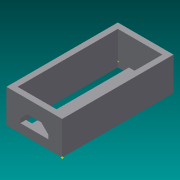
# Autodesk Inventor part: nano_enclosure
Saved by Autodesk Inventor 2015 (Build 190159000, 159)
## iProperties
Created: 2015-02-05
Part Number: nano_enclosure
Material: Generic
Document SubType Name: Modeling
Designer: Jeff
Density: 1 g/cm^3
Appearance: Default
Author: Jeff
Autodesk Inventor part; units mm, degrees
ref_plane "YZ Plane" through (0, 0, 0) normal (1, 0, 0) x (0, 1, 0)
ref_plane "XZ Plane" through (0, 0, 0) normal (0, 1, 0) x (-1, 0, 0)
ref_plane "XY Plane" through (0, 0, 0) normal (0, 0, 1) x (1, 0, 0)
sketch "Sketch1" plane through (0, 0, 0) normal (0, 1, 0) x (-1, 0, 0)
  line L0 (0, 0) -> (25.4, 0)
  line L1 (25.4, 0) -> (25.4, -50.8)
  line L2 (25.4, -50.8) -> (0, -50.8)
  line L3 (0, -50.8) -> (0, 0)
  dimension "d0" = 25.4
  dimension "d1" = 50.8
  constraints: 8 end point, 2 parallel, 1 horizontal, 1 perpendicular
  measures "d0" distance of L1.end L2.end
  measures "d1" distance of L0.end L1.end
extrude "Extrusion1" add sketch "Sketch1" along normal blind 15.24
shell "Shell1" thickness 2.54 removed faces 1 at (-8.4667, 15.24, -33.8667)
sketch "Sketch3" plane through (-25.4, 0, 0) normal (0, 0, 1) x (1, 0, 0)
  line L0 (19.05, 4.064) -> (6.35, 4.064)
  line L1 (6.35, 4.064) -> (6.35, 9.144)
  line L2 (6.35, 9.144) -> (19.05, 9.144)
  line L3 (19.05, 9.144) -> (19.05, 4.064)
  point P0 (25.4, 0)
  dimension "d20" = 4.064
  dimension "d21" = 12.7
  dimension "d22" = 5.08
  dimension "d23" = 6.35
  constraints: 8 end point, 2 parallel, 1 horizontal, 1 perpendicular
  measures "d20" distance from line of point (25.4, 0) L0
  measures "d21" distance of L1.end L2.end
  measures "d22" distance of L2.end L0.start
  measures "d23" distance from line of point (25.4, 0) L3
extrude "Extrusion3" cut sketch "Sketch3" against normal blind 2.54
chamfer "Chamfer1" distance 3.175 angle 45 2 edges at (-19.05, 9.144, -1.27) (-6.35, 9.144, -1.27)
sketch "Sketch5" plane through (-22.86, 2.54, -2.54) normal (0, 1, 0) x (1, 0, 0)
  line L0 (0, 0) -> (5.08, 0)
  line L1 (5.08, 0) -> (5.08, 45.72)
  line L2 (5.08, 45.72) -> (0, 45.72)
  line L3 (0, 45.72) -> (0, 0)
  line L4 (0, 45.72) -> (20.32, 45.72) projected
  line L5 (20.32, 0) -> (15.24, 0)
  line L6 (15.24, 0) -> (15.24, 45.72)
  line L7 (15.24, 45.72) -> (20.32, 45.72)
  line L8 (20.32, 45.72) -> (20.32, 0)
  point P0 (22.86, -2.54)
  dimension "d29" = 5.08
  dimension "d30" = 5.08
  constraints: 16 end point, 4 parallel, 2 coincident, 2 horizontal, 2 perpendicular, 1 point on line
  measures "d29" distance between parallel lines of L1 L3
  measures "d30" distance between parallel lines of L8 L6
extrude "Extrusion4" cut sketch "Sketch5" against normal blind 2.54
body "Solid1"
